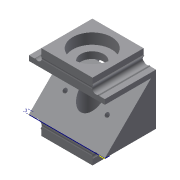
# Autodesk Inventor part: 20_Cube_Insert_Beamsplitter
Saved by Autodesk Inventor 2019 (Build 230136000, 136)
## iProperties
Created: 2019-08-06
Part Number: 20_Cube_Insert_Beamsplitter
Material: Generic
Document SubType Name: Modeling
Designer: marsikovabarbora
Density: 1 g/cm^3
Appearance: Default
Author: marsikovabarbora
Autodesk Inventor part; units mm, degrees
ref_plane "YZ Plane" through (0, 0, 0) normal (1, 0, 0) x (0, 1, 0)
sketch "Sketch1" plane through (0, 0, 0) normal (0, 0, 1) x (1, 0, 0)
  line L0 (-34.86, 0) -> (34.86, 0) construction
  line L1 (0, -34.86) -> (0, 34.86) construction
  line L2 (0, 0) -> (16.9726, 16.9726) construction
  line L3 (0, 0) -> (24.0028, 0) construction
  line L4 (0, 24.9) -> (16.8009, 24.9)
  line L5 (16.8009, 24.9) -> (16.8009, 21.2415)
  line L6 (16.8009, 21.2415) -> (19.0212, 19.0212)
  line L7 (24.9, 0) -> (24.9, 16.8009)
  line L8 (24.9, 16.8009) -> (21.2415, 16.8009)
  line L9 (21.2415, 16.8009) -> (19.0212, 19.0212)
  line L10 (0, -24.9) -> (16.8009, -24.9)
  line L11 (16.8009, -24.9) -> (16.8009, -21.2415)
  line L12 (16.8009, -21.2415) -> (19.0212, -19.0212)
  line L13 (24.9, 0) -> (24.9, -16.8009)
  line L14 (24.9, -16.8009) -> (21.2415, -16.8009)
  line L15 (21.2415, -16.8009) -> (19.0212, -19.0212)
  line L16 (0, 0) -> (-16.9726, 16.9726) construction
  line L17 (0, 0) -> (-24.0028, 0) construction
  line L18 (0, 24.9) -> (-16.8009, 24.9)
  line L19 (-16.8009, 24.9) -> (-16.8009, 21.2415)
  line L20 (-16.8009, 21.2415) -> (-19.0212, 19.0212)
  line L21 (-24.9, 0) -> (-24.9, 16.8009)
  line L22 (-24.9, 16.8009) -> (-21.2415, 16.8009)
  line L23 (-21.2415, 16.8009) -> (-19.0212, 19.0212)
  line L24 (0, -24.9) -> (-16.8009, -24.9)
  line L25 (-16.8009, -24.9) -> (-16.8009, -21.2415)
  line L26 (-16.8009, -21.2415) -> (-19.0212, -19.0212)
  line L27 (-21.2415, -16.8009) -> (-19.0212, -19.0212)
  line L28 (-24.9, -16.8009) -> (-21.2415, -16.8009)
  line L29 (-24.9, 0) -> (-24.9, -16.8009)
  circle A0 centre (0, 0) radius 7.5
  dimension "d17" = 45
  dimension "d18" = 24.9
  dimension "d20" = 3.14
  dimension "d21" = 26.9
  dimension "d22" = 15
  constraints: 56 end point, 22 symmetric about line, 3 point on line, 2 horizontal, 2 perpendicular, 1 centre point, 1 coincident, 1 equal length
  measures "d17" angle of L3 L2
  measures "d18" distance between parallel lines of L0 L4
  measures "d20" distance of L5.end L6.end
  measures "d21" distance from line of L2.start L6
  measures "d22" diameter of A0
extrude "Extrusion1" add sketch "Sketch1" along normal blind 3
sketch "Sketch6" plane through (0, 0, 3) normal (0, 0, 1) x (1, 0, 0)
  circle A0 centre (0, 0) radius 7.5 projected
  line L0 (16.8009, 24.9) -> (-16.8009, 24.9) projected
  line L1 (-16.8009, 24.9) -> (-16.8009, 21.2415) projected
  line L2 (-16.8009, 21.2415) -> (-21.2415, 16.8009) projected
  line L3 (-21.2415, 16.8009) -> (-24.9, 16.8009) projected
  line L4 (-24.9, 16.8009) -> (-24.9, -16.8009) projected
  line L5 (-24.9, -16.8009) -> (-21.2415, -16.8009) projected
  line L6 (-21.2415, -16.8009) -> (-16.8009, -21.2415) projected
  line L7 (-16.8009, -21.2415) -> (-16.8009, -24.9) projected
  line L8 (-16.8009, -24.9) -> (16.8009, -24.9) projected
  line L9 (16.8009, -24.9) -> (16.8009, -21.2415) projected
  line L10 (16.8009, -21.2415) -> (21.2415, -16.8009) projected
  line L11 (21.2415, -16.8009) -> (24.9, -16.8009) projected
  line L12 (24.9, -16.8009) -> (24.9, 16.8009) projected
  line L13 (24.9, 16.8009) -> (21.2415, 16.8009) projected
  line L14 (21.2415, 16.8009) -> (16.8009, 21.2415) projected
  line L15 (16.8009, 21.2415) -> (16.8009, 24.9) projected
  line L16 (24.9, -16.8009) -> (24.9, 16.8009) projected
  line L17 (24.9, 13.5502) -> (-24.9, 13.5502)
  line L18 (-24.9, 16.8009) -> (-24.9, -16.8009) projected
  constraints: 2 end point, 2 point on line, 1 perpendicular
ref_plane "Work Plane2" through (-27.39, -0.0644, 16.8356) normal (0, -0.7071, -0.7071) x (0, 0.7071, -0.7071)
extrude "Extrusion6" add sketch "Sketch6" along normal up to surface contours L12 L11 L10 L9 L8 L7 L6 L5 L4 L17 surface through (-27.39, -0.0644, 16.8356) normal (0, -0.7071, -0.7071)
sketch "Sketch7" plane through (-16.8009, -24.9, 0) normal (0, -1, 0) x (1, 0, 0)
  line L0 (-0.0991, 33.8) -> (0.8009, 33.8) projected
  arc A0 (-6.0991, 41.8) -> (-8.0991, 39.8) centre (-6.0991, 39.8) ccw projected
  arc A1 (41.7009, 39.8) -> (39.7009, 41.8) centre (39.7009, 39.8) ccw projected
  line L1 (41.9057, 41.8) -> (-10.6447, 41.8)
  line L2 (-10.6447, 41.8) -> (-10.6447, 33.8)
  line L3 (-10.6447, 33.8) -> (41.9057, 33.8)
  line L4 (41.9057, 33.8) -> (41.9057, 41.8)
  point P0 (16.8009, 0)
  constraints: 8 end point, 2 parallel, 1 horizontal, 1 perpendicular
extrude "Extrusion7" cut sketch "Sketch7" against normal through all
sketch "Sketch8" plane through (21.2415, -16.8009, 0) normal (0, -1, 0) x (1, 0, 0)
  line L0 (-8.7415, 0) -> (-33.7415, 0) projected
  line L1 (-33.7415, -1) -> (-8.7415, -1) projected
  line L2 (-46.1415, 33.572) -> (-42.483, 33.572) projected
  line L3 (3.6585, 33.8) -> (0.0423, 33.8) projected
  line L4 (0, 33.572) -> (3.6585, 33.572) projected
  line L5 (-46.1415, 3.2209) -> (-46.1415, 33.572) projected
  line L6 (3.6585, 33.572) -> (-46.1415, 33.572)
  line L7 (-46.1415, 33.572) -> (-46.1415, 30.572)
  line L8 (-46.1415, 30.572) -> (3.6585, 30.572)
  line L9 (3.6585, 30.572) -> (3.6585, 33.572)
  dimension "d45" = 3
  constraints: 8 end point, 2 parallel, 1 horizontal, 1 perpendicular, 1 point on line
  measures "d45" distance of L7.end L6.end
sketch "Sketch9" plane through (-16.8009, -24.9, 0) normal (0, -1, 0) x (1, 0, 0)
  line L0 (33.7009, 0) -> (33.0009, 0) construction
  line L1 (36.0327, -6) -> (22.7009, -6) construction
  circle A0 centre (16.8009, 16.9) radius 16.9 construction
  circle A1 centre (16.8009, 16.9) radius 7.5
  line L2 (39.7009, 8.1978) -> (33.7009, 8.1978) projected
  line L3 (33.7009, 8.1978) -> (33.7009, 0) projected
  line L4 (33.0009, 0) -> (33.0009, -3.7) projected
  line L5 (33.0009, -3.7) -> (22.7009, -3.7) projected
  line L6 (22.7009, -3.7) -> (22.7009, -6) projected
  arc A2 (39.7009, -2.3319) -> (36.0327, -6) centre (36.8009, -3.1) ccw projected
  line L7 (39.7009, 8.1978) -> (39.7009, -2.3319) projected
  point P0 (16.8009, 0)
  dimension "d46" = 15
  constraints: 2 centre point, 1 coincident, 1 tangent
  measures "d46" diameter of A1
extrude "Extrusion8" cut sketch "Sketch9" against normal through all
sketch "Sketch10" plane through (-16.8009, -24.9, 0) normal (0, -1, 0) x (1, 0, 0)
  circle A0 centre (16.8009, 16.9) radius 7.5 projected
  circle A1 centre (16.8009, 16.9) radius 12.75
  point P0 (16.8009, 0)
  dimension "d49" = 25.5
  constraints: 1 centre point, 1 coincident
  measures "d49" diameter of A1
extrude "Extrusion9" cut sketch "Sketch10" against normal blind 7
sketch "Sketch11" plane through (0, 0, 0) normal (0, 0, -1) x (-1, 0, 0)
  circle A0 centre (0, 0) radius 7.5 projected
  circle A1 centre (0, 0) radius 12.75
  dimension "d52" = 25.5
  constraints: 1 centre point, 1 coincident
  measures "d52" diameter of A1
extrude "Extrusion10" cut sketch "Sketch11" against normal blind 7
sketch "Sketch12" plane through (-24.9, 13.5502, 3.2209) normal (0, 0.7071, 0.7071) x (1, 0, 0)
  line L0 (32.9, -31.2053) -> (32.9, -6.2053) construction
  line L1 (32.9, -6.2053) -> (16.9, -6.2053) construction
  line L2 (16.9, -6.2053) -> (16.9, -31.2053) construction
  line L3 (16.9, -31.2053) -> (32.9, -31.2053) construction
  line L4 (37.7, -37.554) -> (12.1, -37.554)
  line L5 (12.1, -37.554) -> (12.1, -0.954)
  line L6 (12.1, -0.954) -> (37.7, -0.954)
  line L7 (37.7, -0.954) -> (37.7, -37.554)
  line L8 (17.4003, -19.254) -> (32.3997, -19.254) projected
  line L9 (37.7, -37.554) -> (12.1, -0.954) construction
  line L10 (12.1, -37.554) -> (37.7, -0.954) construction
  line L11 (10.6, -39.054) -> (39.2, -39.054)
  line L12 (39.2, -39.054) -> (39.2, 0.546)
  line L13 (39.2, 0.546) -> (10.6, 0.546)
  line L14 (10.6, 0.546) -> (10.6, -39.054)
  point P0 (24.9, -19.254)
  dimension "d81" = 25.6
  dimension "d82" = 36.6
  dimension "d83" = 1.5
  constraints: 20 end point, 4 parallel, 3 midpoint, 2 perpendicular, 1 horizontal, 3 other
  measures "d81" distance of L5.end L6.end
  measures "d82" distance of L4.end L5.end
  measures "d83" distance between parallel lines of L4 L11
extrude "Extrusion11" add sketch "Sketch12" along normal blind 1
sketch "Sketch13" plane through (0, 0, 3) normal (0, 0, 1) x (1, 0, 0)
  line L0 (-24.9, 13.5502) -> (24.9, 13.5502) projected
  line L1 (24.9, 13.5502) -> (24.9, 16.8009) projected
  line L2 (24.9, 16.8009) -> (21.2415, 16.8009) projected
  line L3 (21.2415, 16.8009) -> (16.8009, 21.2415) projected
  line L4 (16.8009, 21.2415) -> (16.8009, 24.9) projected
  line L5 (16.8009, 24.9) -> (-16.8009, 24.9) projected
  line L6 (-16.8009, 24.9) -> (-16.8009, 21.2415) projected
  line L7 (-16.8009, 21.2415) -> (-21.2415, 16.8009) projected
  line L8 (-21.2415, 16.8009) -> (-24.9, 16.8009) projected
  line L9 (-24.9, 16.8009) -> (-24.9, 13.5502) projected
  point P0 (0, 0)
ref_plane "Work Plane3" through (-16.9, 21.1423, 33.8) normal (0, 0, -1) x (0, 1, 0)
extrude "Extrusion12" add sketch "Sketch13" along normal up to surface (30.8 mm away)
sketch "Sketch14" plane through (-16.8009, 24.9, 0) normal (0, 1, 0) x (1, 0, 0)
  line L0 (-0.0991, -33.8) -> (-0.0991, 0) construction
  line L1 (33.6017, -33.8) -> (0, -33.8) projected
  line L2 (0, 0) -> (33.6017, 0) projected
  line L3 (33.6017, 0) -> (33.6017, -33.8) projected
  arc A0 (9.3011, -16.8356) -> (24.3006, -16.8356) centre (16.8009, -16.9) ccw construction
  circle A1 centre (16.8009, -16.9) radius 12.75
  point P0 (16.8009, 0)
  dimension "d61" = 25.5
  constraints: 1 centre point, 1 coincident
  measures "d61" diameter of A1
extrude "Extrusion13" cut sketch "Sketch14" against normal blind 7
sketch "Sketch15" plane through (0, 17.9, 16.9) normal (0, 1, 0) x (1, 0, 0)
  circle A0 centre (0, 0) radius 7.5 projected
  circle A1 centre (0, 0) radius 12
  point P0 (0, 16.9)
  dimension "d84" = 24
  constraints: 1 centre point, 1 coincident
  measures "d84" diameter of A1
extrude "Extrusion14" cut sketch "Sketch15" against normal through all contours A0 | A1
sketch "Sketch16" plane through (21.2415, -16.8009, 33.572) normal (0, 0.7071, 0.7071) x (1, 0, 0)
  line L0 (-42.255, -0.3224) -> (-0.228, -0.3224) projected
  line L1 (-0.228, -0.3224) -> (0, 0) projected
  line L2 (0, 0) -> (3.6585, 0) projected
  line L3 (3.6585, 0) -> (3.6585, 42.9229) projected
  line L4 (-35.5415, 42.9229) -> (-46.1415, 42.9229) projected
  line L5 (-46.1415, 42.9229) -> (-46.1415, 0) projected
  line L6 (-46.1415, 0) -> (-42.483, 0) projected
  line L7 (-42.483, 0) -> (-42.255, -0.3224) projected
  ellipse E0 centre (-21.2415, 23.76) end of major axis (-21.2415, 41.7912) minor radius 12.75 (-13.0508, 37.5785) -> (-29.4321, 37.5785) ccw projected
  line L8 (-4.4406, 18.0121) -> (-38.0423, 18.0121) projected
  circle A0 centre (-37.2415, 18.0121) radius 1.4
  circle A1 centre (-5.2415, 18.0121) radius 1.4
  line L9 (-13.0508, 37.5785) -> (-14.4599, 37.5785) projected
  line L10 (-35.5415, 3.8689) -> (-35.5415, 42.9229) projected
  line L11 (3.6585, 42.9229) -> (-6.9415, 42.9229) projected
  line L12 (-6.9415, 42.9229) -> (-6.9415, 3.8689) projected
  line L13 (-6.9415, 3.8689) -> (-35.5415, 3.8689) projected
  ellipse E1 centre (-21.2415, 23.5778) end of major axis (-21.2415, 40.5484) minor radius 12 (-28.0231, 37.5785) -> (-14.4599, 37.5785) ccw projected
  line L14 (-28.0231, 37.5785) -> (-29.4321, 37.5785) projected
  point P0 (-21.2415, 35.619)
  dimension "d68" = 2.8
  dimension "d69" = 2.8
  dimension "d85" = 16
  dimension "d86" = 16
  constraints: 4 point on line, 3 coincident, 2 centre point, 2 other
  measures "d68" diameter of A0
  measures "d69" diameter of A1
  measures "d85" horizontal distance of point (-21.241, 23.578) A1.centre
  measures "d86" horizontal distance of A0.centre point (-21.241, 23.76)
extrude "Extrusion15" cut sketch "Sketch16" along normal through all both and the other way through all contours A1 | A0
sketch "Sketch17" plane through (-24.9, -16.8009, 0) normal (-1, 0, 0) x (0, 0, 1)
  line L0 (43.2726, 50.002) -> (33.5, 50.002)
  line L1 (33.5, 50.002) -> (33.5, -21.818)
  line L2 (33.5, -21.818) -> (43.2726, -21.818)
  line L3 (43.2726, -21.818) -> (43.2726, 50.002)
  line L4 (0, 0) -> (0, 33.6017) projected
  point P0 (0, 16.8009)
  dimension "d72" = 33.5
  constraints: 8 end point, 2 parallel, 1 horizontal, 1 perpendicular
  measures "d72" distance between parallel lines of L1 L4
extrude "Extrusion16" cut sketch "Sketch17" against normal through all
sketch "Sketch18" plane through (-24.9, 13.5502, 33.5) normal (0, 0, 1) x (1, 0, 0)
  line L0 (49.8, 0) -> (0, 0) projected
  line L1 (49.8, 3.2506) -> (49.8, 0) projected
  line L2 (46.1415, 3.2506) -> (49.8, 3.2506) projected
  line L3 (41.7009, 7.6912) -> (46.1415, 3.2506) projected
  line L4 (41.7009, 11.3498) -> (41.7009, 7.6912) projected
  line L5 (8.0991, 11.3498) -> (41.7009, 11.3498) projected
  line L6 (8.0991, 7.6912) -> (8.0991, 11.3498) projected
  line L7 (3.6585, 3.2506) -> (8.0991, 7.6912) projected
  line L8 (0, 3.2506) -> (3.6585, 3.2506) projected
  line L9 (0, 0) -> (0, 3.2506) projected
  line L10 (3.6585, -30.3511) -> (0, -30.3511) projected
  line L11 (8.0991, -34.7917) -> (3.6585, -30.3511) projected
  line L12 (8.0991, -38.4502) -> (8.0991, -34.7917) projected
  line L13 (41.7009, -38.4502) -> (8.0991, -38.4502) projected
  line L14 (41.7009, -34.7917) -> (41.7009, -38.4502) projected
  line L15 (46.1415, -30.3511) -> (41.7009, -34.7917) projected
  line L16 (49.8, -30.3511) -> (46.1415, -30.3511) projected
  line L17 (49.8, -30.2791) -> (49.8, -30.3511) projected
  line L18 (0, -30.2791) -> (49.8, -30.2791) projected
  line L19 (0, -30.3511) -> (0, -30.2791) projected
  line L20 (41.7009, 7.6912) -> (46.1415, 3.2506) construction
  line L21 (43.9212, 5.4709) -> (5.8788, -32.5714) construction
  line L22 (8.0991, -34.7917) -> (3.6585, -30.3511) construction
  circle A0 centre (43.9212, 5.4709) radius 2.5
  point P0 (24.9, -13.5502)
  dimension "d75" = 5
  constraints: 2 end point, 2 midpoint, 1 centre point, 1 coincident
  measures "d75" diameter of A0
extrude "Extrusion17" cut sketch "Sketch18" against normal through all contours A0 L3 | L3 A0
mirror "Mirror3" about plane through (0, 0, 0) normal (1, 0, 0) of "Extrusion17"
mirror "Mirror4" about plane through (0, 0, 0) normal (0, 1, 0) of "Extrusion17", "Mirror3"
pattern_circular "Circular Pattern1" count 4 over 360 about axis through (0, -24.9, 16.9) along (0, 1, 0) of "Extrusion17", "Mirror3", "Mirror4"
sketch "Sketch19" plane through (-12.8, -13.0045, 29.7756) normal (0, 0.7071, 0.7071) x (1, 0, 0)
  line L0 (0, 36.554) -> (-1.5, 36.554) projected
  line L1 (-1.5, 36.554) -> (-1.5, -1.5) projected
  line L2 (-1.5, -1.5) -> (27.1, -1.5) projected
  line L3 (27.1, -1.5) -> (27.1, 36.554) projected
  line L4 (27.1, 36.554) -> (25.6, 36.554) projected
  line L5 (25.6, 36.554) -> (25.6, 0) projected
  line L6 (25.6, 0) -> (0, 0) projected
  line L7 (0, 0) -> (0, 36.554) projected
  line L8 (25.6, 0) -> (25.6, 36.6) projected
  line L9 (0, 0) -> (25.6, 0) projected
  line L10 (0, 36.6) -> (0, 0) projected
  line L11 (25.6, -1.5) -> (0, -1.5)
  line L12 (0, -1.5) -> (0, 36.6)
  line L13 (0, 36.6) -> (25.6, 36.6)
  line L14 (25.6, 36.6) -> (25.6, -1.5)
  line L15 (25.6, -1.5) -> (0, -1.5)
  line L16 (0, -1.5) -> (0, -6.2491)
  line L17 (0, -6.2491) -> (25.6, -6.2491)
  line L18 (25.6, -6.2491) -> (25.6, -1.5)
  point P0 (12.8, 30.2501)
  constraints: 16 end point, 4 parallel, 2 horizontal, 2 perpendicular, 2 point on line
extrude "Extrusion18" cut sketch "Sketch19" along normal mid plane 2 contours L10 L13 L8 L5 L6 L7 | L6 L14 L2 L12 | L2 L18 L17 L16
body "Solid1"
